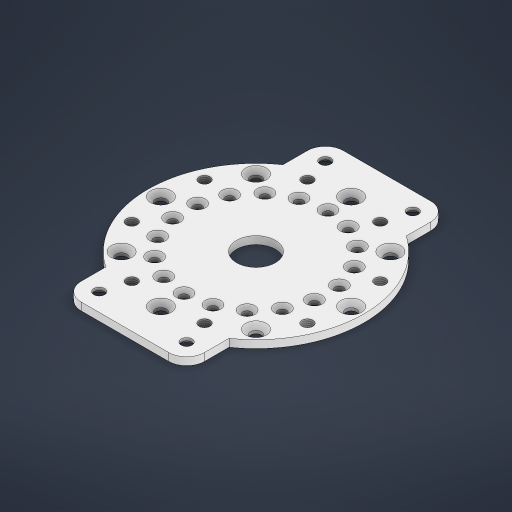
# Autodesk Inventor part: HousingFaceInput
Saved by Autodesk Inventor 2024 (Build 280153000, 153)
## iProperties
Created: 2024-01-31
Part Number: HousingFaceInput
Material: Generic
Document SubType Name: Modeling
Designer: avsar
Density: 1 g/cm^3
Appearance: Smooth - White
Author: avsar
Autodesk Inventor part; units mm, degrees
ref_plane "YZ Plane" through (0, 0, 0) normal (1, 0, 0) x (0, 1, 0)
ref_plane "XZ Plane" through (0, 0, 0) normal (0, 1, 0) x (-1, 0, 0)
ref_plane "XY Plane" through (0, 0, 0) normal (0, 0, 1) x (1, 0, 0)
sketch "Sketch1" plane through (0, 0, 0) normal (0, 1, 0) x (-1, 0, 0)
  circle A0 centre (0, 0) radius 42
  circle A1 centre (0, -28) radius 1.6
  circle A2 centre (0, -28) radius 4.1 construction
  circle A3 centre (9.5766, -26.3114) radius 1.6
  circle A4 centre (17.9981, -21.4492) radius 1.6
  circle A5 centre (24.2487, -14) radius 1.6
  circle A6 centre (27.5746, -4.8621) radius 1.6
  circle A7 centre (27.5746, 4.8621) radius 1.6
  circle A8 centre (24.2487, 14) radius 1.6
  circle A9 centre (17.9981, 21.4492) radius 1.6
  circle A10 centre (9.5766, 26.3114) radius 1.6
  circle A11 centre (0, 28) radius 1.6
  circle A12 centre (-9.5766, 26.3114) radius 1.6
  circle A13 centre (-17.9981, 21.4492) radius 1.6
  circle A14 centre (-24.2487, 14) radius 1.6
  circle A15 centre (-27.5746, 4.8621) radius 1.6
  circle A16 centre (-27.5746, -4.8621) radius 1.6
  circle A17 centre (-24.2487, -14) radius 1.6
  circle A18 centre (-17.9981, -21.4492) radius 1.6
  circle A19 centre (-9.5766, -26.3114) radius 1.6
  circle A20 centre (0, 0) radius 7.55
  circle A21 centre (9.5766, -26.3114) radius 4.1 construction
  circle A22 centre (0, -37) radius 2.1
  circle A23 centre (0, -37) radius 4 construction
  circle A24 centre (14.1593, -34.1835) radius 2.1
  circle A25 centre (26.163, -26.163) radius 2.1
  circle A26 centre (34.1835, -14.1593) radius 2.1
  circle A27 centre (37, 0) radius 2.1
  circle A28 centre (34.1835, 14.1593) radius 2.1
  circle A29 centre (26.163, 26.163) radius 2.1
  circle A30 centre (14.1593, 34.1835) radius 2.1
  circle A31 centre (0, 37) radius 2.1
  circle A32 centre (-14.1593, 34.1835) radius 2.1
  circle A33 centre (-26.163, 26.163) radius 2.1
  circle A34 centre (-34.1835, 14.1593) radius 2.1
  circle A35 centre (-37, 0) radius 2.1
  circle A36 centre (-34.1835, -14.1593) radius 2.1
  circle A37 centre (-26.163, -26.163) radius 2.1
  circle A38 centre (-14.1593, -34.1835) radius 2.1
  dimension "d0" = 84
  dimension "d1" = 3.2
  dimension "d2" = 28
  dimension "d5" = 8.2
  dimension "d8" = 360
  dimension "d14" = 15.1
  dimension "d25" = 8.2
  dimension "d26" = 4.2
  dimension "d27" = 37
  dimension "d28" = 8
  dimension "d31" = 360
  constraints: 39 centre point, 5 coincident, 2 vertical alignment, 70 other
  measures "d0" diameter of A0
  measures "d1" diameter of A1
  measures "d2" distance of point (0, 0) A1.centre
  measures "d5" diameter of A2
  measures "d14" diameter of A20
  measures "d25" diameter of A21
  measures "d26" diameter of A22
  measures "d27" distance of point (0, 0) A22.centre
  measures "d28" diameter of A23
extrude "Extrusion1" add sketch "Sketch1" against normal blind 3 contours A0 | A22 | A24 | A25 | A26 | A27 | A28 | A29 | A30 | A31 | A32 | A33 | A34 | A35 | A36 | A37 | A38
hole "Hole3" at (-17.9981, 0, 21.4492) at (-24.2487, 0, 14) at (-27.5746, 0, 4.8621) at (-27.5746, 0, -4.8621) at (-24.2487, 0, -14) at (-17.9981, 0, -21.4492) at (-9.5766, 0, -26.3114) at (0, 0, -28) at (9.5766, 0, -26.3114) at (17.9981, 0, -21.4492) at (24.2487, 0, -14) at (27.5746, 0, -4.8621) at (27.5746, 0, 4.8621) at (24.2487, 0, 14) at (17.9981, 0, 21.4492) at (9.5766, 0, 26.3114) at (0, 0, 28) at (-9.5766, 0, 26.3114) direction (0, -1, 0) diameter 3.2 end through all countersink diameter 6 countersink angle 90
extrude "Extrusion2" cut sketch "Sketch1" against normal up to surface (3 mm away) contours A24 | A26 | A28 | A30 | A32 | A34 | A36 | A38
thread "Thread1" size "M4.5x0.75" class "6H" standard "ANSI Metric M Profile" full length
thread "Thread2" size "M4.5x0.75" class "6H" standard "ANSI Metric M Profile" full length
thread "Thread3" size "M4.5x0.75" class "6H" standard "ANSI Metric M Profile" full length
thread "Thread4" size "M4.5x0.75" class "6H" standard "ANSI Metric M Profile" full length
thread "Thread5" size "M4.5x0.75" class "6H" standard "ANSI Metric M Profile" full length
thread "Thread6" size "M4.5x0.75" class "6H" standard "ANSI Metric M Profile" full length
thread "Thread7" size "M4.5x0.75" class "6H" standard "ANSI Metric M Profile" full length
thread "Thread8" size "M4.5x0.75" class "6H" standard "ANSI Metric M Profile" full length
sketch "Sketch2" plane through (0, 0, 0) normal (0, 1, 0) x (1, 0, 0)
  line L0 (-24, -51) -> (24, -51)
  line L1 (24, -51) -> (24, -34.4674)
  line L2 (24, 51) -> (-24, 51)
  line L3 (-24, 51) -> (-24, 34.4674)
  circle A0 centre (0, 0) radius 7.55 construction
  line L4 (-24, -51) -> (24, 51) construction
  line L5 (24, -51) -> (-24, 51) construction
  circle A1 centre (0, 0) radius 42 construction
  arc A2 (24, 34.4674) -> (-24, 34.4674) centre (0, 0) ccw
  arc A3 (-24, -34.4674) -> (24, -34.4674) centre (0, 0) ccw
  line L6 (-24, -34.4674) -> (-24, -51)
  line L7 (-24, 34.4674) -> (-24, -34.4674) construction
  line L8 (24, 34.4674) -> (24, 51)
  line L9 (24, -34.4674) -> (24, 34.4674) construction
  dimension "d65" = 48
  dimension "d66" = 102
  constraints: 20 end point, 10 parallel, 8 point on circle, 3 perpendicular, 2 centre point, 2 concentric, 2 midpoint, 1 horizontal
  measures "d65" distance of L2.end L2.start
  measures "d66" distance of L2.start L0.end
extrude "Extrusion3" add sketch "Sketch2" against normal up to surface (3 mm away)
fillet "Fillet1" radius 7 4 edges at (-24, -1.5, 51) (24, -1.5, 51) (24, -1.5, -51) (-24, -1.5, -51)
sketch "Sketch3" plane through (0, 0, 0) normal (0, 1, 0) x (1, 0, 0)
  circle A0 centre (-17, 44) radius 2.1
  arc A1 (-17, 51) -> (-24, 44) centre (-17, 44) ccw construction
  circle A2 centre (17, 44) radius 2.1
  arc A3 (24, 44) -> (17, 51) centre (17, 44) ccw construction
  circle A4 centre (-17, -44) radius 2.1
  circle A5 centre (17, -44) radius 2.1
  arc A6 (-24, -44) -> (-17, -51) centre (-17, -44) ccw construction
  arc A7 (17, -51) -> (24, -44) centre (17, -44) ccw construction
  point P0 (0, 0)
  dimension "d70" = 4.2
  dimension "d71" = 4.2
  dimension "d72" = 4.2
  dimension "d73" = 4.2
  constraints: 4 centre point, 4 concentric
  measures "d70" diameter of A0
  measures "d71" diameter of A2
  measures "d72" diameter of A4
  measures "d73" diameter of A5
extrude "Extrusion4" cut sketch "Sketch3" against normal through all
sketch "Sketch4" plane through (0, -3, 0) normal (0, -1, 0) x (1, 0, 0)
  circle A0 centre (17, 44) radius 2.1 projected
  circle A1 centre (-17, 44) radius 2.1 projected
  circle A2 centre (-17, -44) radius 2.1 projected
  circle A3 centre (17, -44) radius 2.1 projected
  point P0 (0, 0)
hole "Hole4" at (-17, -3, 44) at (17, -3, 44) at (17, -3, -44) at (-17, -3, -44) direction (0, 1, 0) diameter 4.2 end through all countersink diameter 8 countersink angle 90
hole "Hole5" at (-26.163, 0, 26.163) at (-37, 0, 0) at (-26.163, 0, -26.163) at (0, 0, -37) at (26.163, 0, -26.163) at (37, 0, 0) at (26.163, 0, 26.163) at (0, 0, 37) direction (0, -1, 0) diameter 4.2 end through all countersink diameter 8 countersink angle 90
body "Solid1"
